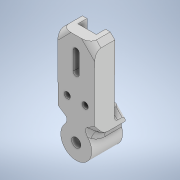
# Autodesk Inventor part: arm_linkage_2
Saved by Autodesk Inventor 2020 (Build 240168000, 168)
## iProperties
Created: 2019-10-19
Part Number: arm_linkage_2
Material: Generic
Document SubType Name: Modeling
Designer: psrob
Density: 1 g/cm^3
Appearance: Default
Author: psrob
Autodesk Inventor part; units mm, degrees
ref_plane "YZ Plane" through (0, 0, 0) normal (1, 0, 0) x (0, 1, 0)
ref_plane "XZ Plane" through (0, 0, 0) normal (0, 1, 0) x (-1, 0, 0)
ref_plane "XY Plane" through (0, 0, 0) normal (0, 0, 1) x (1, 0, 0)
sketch "Sketch1" plane through (0, 0, 0) normal (0, 0, 1) x (1, 0, 0)
  circle A0 centre (5, 51.5563) radius 1.5 projected
  circle A1 centre (5, 51.5563) radius 1.5
  circle A2 centre (5, 51.5563) radius 7.5
  line L0 (5, 51.5563) -> (5, 71.5563)
  line L1 (5, 71.5563) -> (-2.5, 71.5563)
  line L2 (-2.5, 71.5563) -> (12.5, 71.5563)
  line L3 (12.5, 71.5563) -> (12.5, 51.5563)
  line L4 (12.5, 51.5563) -> (-2.5, 51.5563)
  line L5 (-2.5, 51.5563) -> (-2.5, 71.5563)
  point P0 (0, 0)
  point P1 (12.5, 51.5563)
  dimension "d0" = 3
  dimension "d1" = 15
  dimension "d2" = 20
  dimension "d3" = 7.5
  dimension "d4" = 15
  dimension "d5" = 20
  constraints: 12 end point, 2 centre point, 2 coincident, 2 horizontal, 2 parallel, 1 perpendicular, 1 vertical
  measures "d0" diameter of A1
  measures "d1" diameter of A2
  measures "d2" distance of L0.start L0.end
  measures "d3" distance of L0.end L1.end
  measures "d4" distance of L3.end L4.end
  measures "d5" distance of L2.end L3.end
extrude "Extrusion1" add sketch "Sketch1" along normal blind 10 contours L4 A2 A0 | A0 L0 A2 L4 | A0 L4 A2 L0 | A2 L0 L2 L3 | A2 L5 L1 L0
sketch "Sketch2" plane through (0, 0, 10) normal (0, 0, 1) x (1, 0, 0)
  line L0 (-2.5, 71.5563) -> (-2.5, 51.5563) projected
  arc A0 (-2.5, 51.5563) -> (12.5, 51.5563) centre (5, 51.5563) ccw projected
  line L1 (12.5, 51.5563) -> (12.5, 71.5563) projected
  line L2 (12.5, 71.5563) -> (-2.5, 71.5563) projected
  circle A1 centre (5, 51.5563) radius 1.5 projected
  circle A2 centre (5, 51.5563) radius 5
  line L3 (12.5, 71.5563) -> (12.5, 56.5563)
  line L4 (12.5, 51.5563) -> (12.5, 71.5563) projected
  line L5 (12.5, 56.5563) -> (5, 51.5563)
  line L6 (-2.5, 71.5563) -> (-2.5, 56.5563)
  line L7 (-2.5, 71.5563) -> (-2.5, 51.5563) projected
  line L8 (-2.5, 56.5563) -> (5, 51.5563)
  point P0 (0, 0)
  point P1 (9.1603, 54.3299)
  point P2 (0.8397, 54.3299)
  dimension "d8" = 10
  dimension "d9" = 15
  dimension "d10" = 15
  constraints: 8 end point, 2 point on line, 1 centre point, 1 coincident
  measures "d8" diameter of A2
  measures "d9" distance of L1.end L3.end
  measures "d10" distance of L0.start L6.end
extrude "Extrusion2" cut sketch "Sketch2" against normal blind 10 contours L8 A2 L5 L1 A0 L0
thicken "Thicken1" operation add thickness 10 both sides no extend neighbours yes toward (0, 1, 0) faces at (7.5, 71.5563, 3.3333)
sketch "Sketch3" plane through (0, 0, 0) normal (0, 0, -1) x (-1, 0, 0)
  line L0 (-2, 186.5563) -> (-2, 66.5563) projected
  line L1 (-8, 186.5563) -> (-8, 66.5563) projected
  line L2 (-2, 66.5563) -> (-8, 66.5563) projected
  line L3 (-12.5, 81.5563) -> (2.5, 81.5563) projected
  point P0 (0, 0)
  point P1 (-2, 81.5563)
  point P2 (-8, 81.5563)
ref_plane "Work Plane1" through (-40.8822, 64.4122, 6.5) normal (0, 0, 1) x (1, 0, 0)
extrude "Extrusion3" cut sketch "Sketch3" against normal up to surface (6.5 mm away)
sketch "Sketch4" plane through (0, 0, 0) normal (0, 0, -1) x (-1, 0, 0)
  circle A0 centre (-5, 51.5563) radius 1.5 projected
  line L0 (-2, 81.5563) -> (-2, 66.5563) projected
  line L1 (-2, 66.5563) -> (-8, 66.5563) projected
  line L2 (-8, 66.5563) -> (-8, 81.5563) projected
  line L3 (-12.5, 81.5563) -> (-8, 81.5563) projected
  line L4 (-12.5, 56.5563) -> (-12.5, 81.5563) projected
  line L5 (-12.5, 56.5563) -> (-9.1603, 54.3299) projected
  arc A1 (-9.1603, 54.3299) -> (-0.8397, 54.3299) centre (-5, 51.5563) ccw projected
  line L6 (-0.8397, 54.3299) -> (2.5, 56.5563) projected
  line L7 (2.5, 81.5563) -> (2.5, 56.5563) projected
  line L8 (-2, 81.5563) -> (2.5, 81.5563) projected
  line L9 (2.5, 81.5563) -> (1, 81.5563)
  line L10 (-12.5, 81.5563) -> (2.5, 81.5563) projected
  line L11 (1, 81.5563) -> (0.8301, 55.4431)
  line L12 (-0.8397, 54.3299) -> (2.5, 56.5563) projected
  line L13 (-12.5, 56.5563) -> (-12.5, 81.5563) projected
  line L14 (-12.5, 81.5563) -> (-11, 81.5563)
  line L15 (-11, 81.5563) -> (-10.8301, 55.4431)
  line L16 (-12.5, 56.5563) -> (-9.1603, 54.3299) projected
  point P0 (0, 0)
  dimension "d21" = 1.5
  dimension "d22" = 1.5
  constraints: 8 end point, 2 midpoint, 2 point on line
  measures "d21" distance of L7.start L9.end
  measures "d22" distance of L3.start L14.end
extrude "Extrusion4" cut sketch "Sketch4" against normal blind 10 contours L8 L7 L6 L11 | L15 L5 L4 L3
sketch "Sketch5" plane through (0, 0, 0) normal (0, 0, -1) x (-1, 0, 0)
  circle A0 centre (-5, 51.5563) radius 1.5 projected
  line L0 (0.8301, 55.4431) -> (1, 81.5563) projected
  line L1 (-2, 81.5563) -> (1, 81.5563) projected
  line L2 (-2, 81.5563) -> (-2, 66.5563) projected
  line L3 (-2, 66.5563) -> (-8, 66.5563) projected
  line L4 (-8, 66.5563) -> (-8, 81.5563) projected
  line L5 (-11, 81.5563) -> (-8, 81.5563) projected
  line L6 (-11, 81.5563) -> (-10.8301, 55.4431) projected
  line L7 (-10.8301, 55.4431) -> (-9.1603, 54.3299) projected
  arc A1 (-9.1603, 54.3299) -> (-0.8397, 54.3299) centre (-5, 51.5563) ccw projected
  line L8 (-0.8397, 54.3299) -> (0.8301, 55.4431) projected
  circle A2 centre (-5, 51.5563) radius 1.5 projected
  circle A3 centre (-5, 51.5563) radius 7.5
  point P0 (0, 0)
  point P1 (-10.8355, 56.2677)
  point P2 (0.8355, 56.2677)
  dimension "d25" = 15
  constraints: 1 centre point, 1 coincident
  measures "d25" diameter of A3
extrude "Extrusion5" cut sketch "Sketch5" against normal blind 0.5 contours A3 L6 L5 L4 L3 L2 L1 L0
chamfer "Chamfer3" distance 3 angle 45 2 edges at (9.9952, 54.8865, 10) (0.0048, 54.8865, 10)
fillet "Fillet2" radius 4 2 edges at (9.9952, 54.8865, 7) (0.0048, 54.8865, 7)
fillet "Fillet3" radius 1.5 6 edges at (8.9947, 54.5634, 6.8287) (7.5826, 55.8377, 9.1297) (9.1603, 54.3299, 2.6716) (1.0053, 54.5634, 6.8287) (2.4174, 55.8377, 9.1297) (0.8397, 54.3299, 2.6716)
thicken "Thicken2" operation add thickness 3 both sides no extend neighbours yes toward (0, 0, 1) faces at (9.9452, 68.1268, 0.5)
sketch "Sketch6" plane through (8, 66.5563, 3.5) normal (0, 0, -1) x (-1, 0, 0)
  line L0 (9, 15) -> (8.8355, -10.2886) projected
  line L1 (6, 15) -> (9, 15) projected
  line L2 (6, 0) -> (6, 15) projected
  line L3 (0, 0) -> (6, 0) projected
  line L4 (0, 15) -> (0, 0) projected
  line L5 (-3, 15) -> (0, 15) projected
  line L6 (-2.8355, -10.2886) -> (-3, 15) projected
  line L7 (-2.8355, -10.2886) -> (-2.8301, -11.1132) projected
  line L8 (-2.8301, -11.1132) -> (-2.2623, -11.4918) projected
  arc A0 (-1.688, -13.2614) -> (-2.2623, -11.4918) centre (-3.0944, -12.7398) ccw projected
  arc A1 (-1.688, -13.2614) -> (7.688, -13.2614) centre (3, -15) ccw projected
  arc A2 (8.2623, -11.4918) -> (7.688, -13.2614) centre (9.0944, -12.7398) ccw projected
  line L9 (8.2623, -11.4918) -> (8.8301, -11.1132) projected
  line L10 (8.8301, -11.1132) -> (8.8355, -10.2886) projected
  circle A3 centre (3, -15) radius 1.5 projected
  line L11 (-2.8654, -5.6942) -> (-3, 15) projected
  line L12 (-2.8654, -5.6942) -> (-2.8816, -3.1943)
  line L13 (-2.8816, -3.1943) -> (0.1183, -3.1748)
  line L14 (8.8654, -5.6942) -> (8.8816, -3.1943)
  line L15 (9, 15) -> (8.8654, -5.6942) projected
  line L16 (8.8816, -3.1943) -> (5.8817, -3.1748)
  circle A4 centre (0.1183, -3.1748) radius 1
  circle A5 centre (5.8817, -3.1748) radius 1
  arc A6 (8.8355, -10.2886) -> (-2.8355, -10.2886) centre (3, -15) ccw projected
  arc A7 (8.8355, -10.2886) -> (-2.8355, -10.2886) centre (3, -15) ccw projected
  point P0 (8, -66.5563)
  dimension "d41" = 2.5
  dimension "d42" = 3
  dimension "d43" = 2.5
  dimension "d44" = 3
  dimension "d45" = 2
  dimension "d46" = 2
  constraints: 8 end point, 2 centre point, 2 coincident, 2 perpendicular, 2 point on line
  measures "d41" distance of L11.start L12.end
  measures "d42" distance of L12.end L13.end
  measures "d43" distance of L14.start L14.end
  measures "d44" distance of L14.end L16.end
  measures "d45" diameter of A4
  measures "d46" diameter of A5
extrude "Extrusion6" cut sketch "Sketch6" against normal blind 10 contours A4 | A5
sketch "Sketch7" plane through (0, 0, 0) normal (0, 0, -1) x (-1, 0, 0)
  arc A0 (0.8355, 56.2677) -> (-10.8355, 56.2677) centre (-5, 51.5563) ccw projected
  line L0 (-10.8355, 56.2677) -> (-10.8301, 55.4431) projected
  line L1 (-10.8301, 55.4431) -> (-10.2623, 55.0646) projected
  arc A1 (-9.688, 53.2949) -> (-10.2623, 55.0646) centre (-11.0944, 53.8165) ccw projected
  arc A2 (-9.688, 53.2949) -> (-0.312, 53.2949) centre (-5, 51.5563) ccw projected
  arc A3 (0.2623, 55.0646) -> (-0.312, 53.2949) centre (1.0944, 53.8165) ccw projected
  line L2 (0.2623, 55.0646) -> (0.8301, 55.4431) projected
  line L3 (0.8301, 55.4431) -> (0.8355, 56.2677) projected
  circle A4 centre (-5, 51.5563) radius 1.5 projected
  circle A5 centre (-2.1183, 63.3816) radius 1 projected
  circle A6 centre (-7.8817, 63.3816) radius 1 projected
  line L4 (-10.8355, 56.2677) -> (-11, 81.5563) projected
  arc A7 (0.8355, 56.2677) -> (-10.8355, 56.2677) centre (-5, 51.5563) ccw projected
  line L5 (1, 81.5563) -> (0.8355, 56.2677) projected
  line L6 (-2, 81.5563) -> (1, 81.5563) projected
  line L7 (-2, 66.5563) -> (-2, 81.5563) projected
  line L8 (-8, 66.5563) -> (-2, 66.5563) projected
  line L9 (-8, 81.5563) -> (-8, 66.5563) projected
  line L10 (-11, 81.5563) -> (-8, 81.5563) projected
  arc A8 (0.8355, 56.2677) -> (-10.8355, 56.2677) centre (-5, 51.5563) ccw projected
  line L11 (-5, 59.0563) -> (-10.8536, 59.0563)
  line L12 (-5, 59.0563) -> (0.8536, 59.0563)
  point P0 (0, 0)
  point P1 (-10.8534, 59.0184)
  point P2 (0.8355, 56.2677)
  constraints: 4 end point, 4 point on line, 2 point on circle, 1 tangent
extrude "Extrusion7" add sketch "Sketch7" against normal up to surface (3.5 mm away) contours A0 L12 L5 | A0 L4 L11
chamfer "Chamfer5" distance 2 angle 45 2 edges at (-0.8536, 59.0563, 1.75) (10.8536, 59.0563, 1.75)
chamfer "Chamfer6" distance 1.5 angle 45 2 edges at (11, 81.5563, 6.75) (-1, 81.5563, 6.75)
fillet "Fillet4" radius 2 2 edges at (10.2451, 80.8064, 10) (-0.2451, 80.8064, 10)
fillet "Fillet5" radius 1 2 edges at (0.1529, 58.0564, 3.5) (9.8471, 58.0564, 3.5)
fillet "Fillet6" radius 1 2 edges at (0.1529, 58.0564, 0) (9.8471, 58.0564, 0)
sketch "Sketch8" plane through (8, 66.5563, 6.5) normal (0, 0, -1) x (-1, 0, 0)
  line L0 (0, 0) -> (6, 0) projected
  line L1 (6, 0) -> (6, 15) projected
  line L2 (0, 15) -> (6, 15) projected
  line L3 (0, 15) -> (0, 0) projected
  line L4 (0, 0) -> (6, 0) projected
  line L5 (3, 0) -> (3, 7.5)
  line L6 (3, 4.5) -> (3, 10.5) construction
  line L7 (4, 4.5) -> (4, 10.5)
  line L8 (2, 10.5) -> (2, 4.5)
  arc A0 (2, 4.5) -> (4, 4.5) centre (3, 4.5) ccw
  arc A1 (4, 10.5) -> (2, 10.5) centre (3, 10.5) ccw
  point P0 (8, -66.5563)
  dimension "d60" = 7.5
  dimension "d61" = 3
  dimension "d62" = 2
  constraints: 10 end point, 4 point on circle, 4 tangent, 2 centre point, 2 midpoint, 2 vertical, 1 parallel
  measures "d60" distance of L5.start L5.end
  measures "d61" distance of L5.end L6.end
  measures "d62" diameter of A1
extrude "Extrusion8" cut sketch "Sketch8" against normal blind 10 contours A0 L8 A1 L7
body "Solid1"
